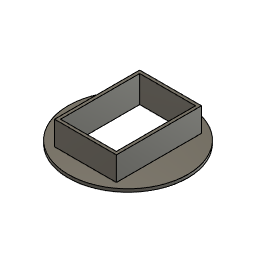
bottom v1 (Autodesk Fusion 360 design; units mm, degrees)
Autodesk Fusion 360 part; units mm, degrees
sketch "Sketch1" plane through (0, 0, 0) normal (0, 1, 0) x (1, 0, 0)
  circle A0 centre (0, 0) radius 40
  line L0 (26.5, -18.7) -> (-26.5, -18.7)
  line L1 (-26.5, -18.7) -> (-26.5, 18.7)
  line L2 (-26.5, 18.7) -> (26.5, 18.7)
  line L3 (26.5, -18.7) -> (-26.5, 18.7) construction
  line L4 (-26.5, -18.7) -> (26.5, 18.7) construction
  line L5 (-28.5, 20.7) -> (28.5, 20.7)
  line L6 (28.5, -20.7) -> (-28.5, -20.7)
  dimension "d1" = 80
  dimension "d2" = 37.4
  dimension "d3" = 53
  dimension "d5" = 37.4
  dimension "d6" = 53
  constraint coincident A0.centre origin
  constraint perpendicular L0 L1
  constraint parallel L0 L2
  constraint horizontal L0
  constraint coincident L3 A0.centre
  constraint coincident L4 A0.centre
  constraint parallel L2 L5
  constraint parallel L0 L6
  measures "d1" diameter of A0
  measures "d2" distance of L0.end L1.end
  measures "d3" distance of L1.end L2.end
  measures "d5" distance of L0.start L2.end
  measures "d6" distance of L1.end L2.end
extrude "Extrude1" add sketch "Sketch1" along normal blind 2
sketch "Sketch2" plane through (0, 2, 0) normal (0, 1, 0) x (-1, 0, 0)
  circle A0 centre (0, 0) radius 40
  line L0 (-18.7, 26.5) -> (18.7, 26.5)
  line L1 (18.7, 26.5) -> (18.7, -26.5)
  line L2 (18.7, -26.5) -> (-18.7, -26.5)
  line L3 (-18.7, -26.5) -> (-18.7, 26.5)
  line L4 (-18.7, 26.5) -> (18.7, -26.5) construction
  line L5 (18.7, 26.5) -> (-18.7, -26.5) construction
  line L6 (20.7, 28.5) -> (20.7, -28.5)
  line L7 (20.7, -28.5) -> (-20.7, -28.5)
  line L8 (-20.7, -28.5) -> (-20.7, 28.5)
  line L9 (-20.7, 28.5) -> (20.7, 28.5)
  dimension "d9" = 37.4
  dimension "d10" = 53
  dimension "d11" = -2
  constraint perpendicular L0 L1
  constraint parallel L0 L2
  constraint parallel L1 L3
  constraint horizontal L0
  constraint coincident L4 A0.centre
  constraint coincident L5 A0.centre
  constraint coincident A0.centre origin
  measures "d9" distance of L1.end L2.end
  measures "d10" distance of L0.end L1.end
extrude "Extrude2" add sketch "Sketch2" along normal blind 16 contours L6 L7 L8 L9
extrude "Extrude3" cut 1 faces at (-6.2333, 2, -8.8333) along direction (0, -1, 0) blind 13
